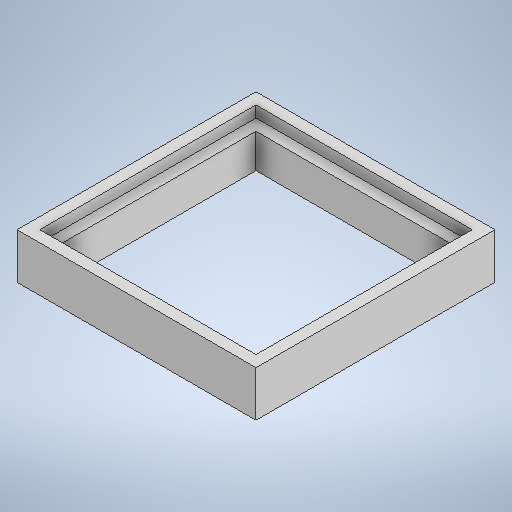
# Autodesk Inventor part: rebord
Saved by Autodesk Inventor 2025.2 (Build 292293000, 293)
## iProperties
Created: 2025-02-16
Part Number: rebord
Material: Générique
Document SubType Name: Modeling
Designer: antoi
Density: 1 g/cm^3
Appearance: Par défaut
Author: antoi
Autodesk Inventor part; units mm, degrees
ref_plane "YZ Plane" through (0, 0, 0) normal (1, 0, 0) x (0, 1, 0)
ref_plane "XZ Plane" through (0, 0, 0) normal (0, 1, 0) x (-1, 0, 0)
ref_plane "XY Plane" through (0, 0, 0) normal (0, 0, 1) x (1, 0, 0)
sketch "Esquisse2" plane through (0, 0, 0) normal (0, 1, 0) x (-1, 0, 0)
  line L0 (0, 0) -> (105, 0)
  line L1 (105, 0) -> (105, -105)
  line L2 (105, -105) -> (0, -105)
  line L3 (0, -105) -> (0, 0)
  line L4 (10, -10) -> (95, -10)
  line L5 (95, -10) -> (95, -95)
  line L6 (95, -95) -> (10, -95)
  line L7 (10, -95) -> (10, -10)
  dimension "d0" = 105
  dimension "d1" = 105
  dimension "d2" = 85
  dimension "d3" = 85
  constraints: 16 end point, 4 parallel, 2 horizontal, 2 perpendicular
  measures "d0" distance of L1.end L2.end
  measures "d1" distance of L0.end L1.end
  measures "d2" distance of L5.end L6.end
  measures "d3" distance of L4.end L5.end
extrude "Extrusion1" add sketch "Esquisse2" along normal blind 20
sketch "Esquisse3" plane through (0, 20, 0) normal (0, 1, 0) x (1, 0, 0)
  line L0 (-95, 10) -> (-95, 95) projected
  line L1 (-10, 10) -> (-95, 10)
  line L2 (-95, 10) -> (-95, 95)
  line L3 (-95, 95) -> (-10, 95)
  line L4 (-10, 95) -> (-10, 10)
  line L5 (-5, 5) -> (-100, 5)
  line L6 (-100, 5) -> (-100, 100)
  line L7 (-100, 100) -> (-5, 100)
  line L8 (-5, 100) -> (-5, 5)
  point P0 (0, 0)
  dimension "d6" = 95
  dimension "d7" = 95
  constraints: 16 end point, 4 parallel, 2 horizontal, 2 perpendicular
  measures "d6" distance of L6.end L7.end
  measures "d7" distance of L5.end L6.end
extrude "Extrusion2" cut sketch "Esquisse3" against normal blind 5
